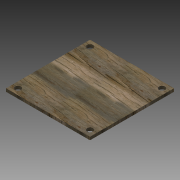
# Autodesk Inventor part: Compact Electric Board
Saved by Autodesk Inventor 2015 (Build 190159000, 159)
## iProperties
Created: 2015-02-05
Part Number: Compact Electric Board
Material: Generic
Document SubType Name: Modeling
Designer: pltwe4
Density: 1 g/cm^3
Appearance: Driftwood
Author: pltwe4
Autodesk Inventor part; units mm, degrees
ref_plane "YZ Plane" through (0, 0, 0) normal (1, 0, 0) x (0, 1, 0)
ref_plane "XZ Plane" through (0, 0, 0) normal (0, 1, 0) x (-1, 0, 0)
ref_plane "XY Plane" through (0, 0, 0) normal (0, 0, 1) x (1, 0, 0)
sketch "Sketch1" plane through (0, 0, 0) normal (0, 1, 0) x (-1, 0, 0)
  line L0 (88.9, 88.9) -> (-88.9, 88.9)
  line L1 (-88.9, 88.9) -> (-88.9, -88.9)
  line L2 (-88.9, -88.9) -> (88.9, -88.9)
  line L3 (88.9, -88.9) -> (88.9, 88.9)
  line L4 (0, -124.46) -> (0, 124.46) projected
  line L5 (-124.46, 0) -> (124.46, 0) projected
  circle A0 centre (76.2, 76.2) radius 6.35
  circle A1 centre (-76.2, 76.2) radius 6.35
  circle A2 centre (-76.2, -76.2) radius 6.35
  circle A3 centre (76.2, -76.2) radius 6.35
  point P0 (0, 0)
  dimension "d0" = 177.8
  dimension "d1" = 177.8
  dimension "d4" = 12.7
  dimension "d5" = 12.7
  dimension "d6" = 12.7
  dimension "d9" = 360
  constraints: 8 end point, 4 centre point, 2 parallel, 1 horizontal, 1 perpendicular, 11 other
  measures "d0" distance of L2.end L0.start
  measures "d1" distance of L1.end L2.end
  measures "d4" diameter of A0
  measures "d5" distance from line of L3 A0.centre
  measures "d6" distance from line of L0 A0.centre
extrude "Extrusion1" add sketch "Sketch1" along normal blind 6.35
body "Solid1"
